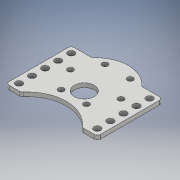
# Autodesk Inventor part: NeverRestMotorMount
Saved by Autodesk Inventor 2018 (Build 220112000, 112)
## iProperties
Created: 2017-11-21
Part Number: NeverRestMotorMount
Material: Generic
Document SubType Name: Modeling
Designer: JM_MRI
Density: 1 g/cm^3
Appearance: Default
Author: JM_MRI
Autodesk Inventor part; units mm, degrees
ref_plane "YZ Plane" through (0, 0, 0) normal (1, 0, 0) x (0, 1, 0)
ref_plane "XZ Plane" through (0, 0, 0) normal (0, 1, 0) x (-1, 0, 0)
ref_plane "XY Plane" through (0, 0, 0) normal (0, 0, 1) x (1, 0, 0)
sketch "Sketch1" plane through (0, 0, 0) normal (0, 0, 1) x (1, 0, 0)
  line L0 (56, 0) -> (56, 40)
  line L1 (0, 40) -> (0, 0)
  circle A0 centre (28, 20) radius 6.1
  circle A1 centre (43.5, 27) radius 1.75
  circle A2 centre (35.75, 40.4234) radius 1.75
  circle A3 centre (20.25, 40.4234) radius 1.75
  circle A4 centre (12.5, 27) radius 1.75
  circle A5 centre (20.25, 13.5766) radius 1.75
  circle A6 centre (35.75, 13.5766) radius 1.75
  arc A7 (43.1987, 40) -> (12.8013, 40) centre (28, 27) ccw
  line L2 (56, 40) -> (43.1987, 40)
  line L3 (12.8013, 40) -> (0, 40)
  circle A8 centre (4, 36) radius 2.05
  circle A9 centre (4, 28) radius 2.05
  circle A10 centre (4, 20) radius 2.05
  circle A11 centre (4, 12) radius 2.05
  circle A12 centre (4, 4) radius 2.05
  circle A13 centre (52, 36) radius 2.05
  circle A14 centre (52, 28) radius 2.05
  circle A15 centre (52, 20) radius 2.05
  circle A16 centre (52, 12) radius 2.05
  circle A17 centre (52, 4) radius 2.05
  arc A18 (46.735, 0) -> (9.265, 0) centre (28, -15) ccw
  line L4 (0, 0) -> (9.265, 0)
  line L5 (46.735, 0) -> (56, 0)
  dimension "d0" = 40
  dimension "d1" = 56
  dimension "d2" = 12.2
  dimension "d4" = 28
  dimension "d5" = 7
  dimension "d6" = 15.5
  dimension "d7" = 3.5
  dimension "d10" = 360
  dimension "d12" = 20
  dimension "d14" = 20
  dimension "d15" = 4.1
  dimension "d16" = 4
  dimension "d17" = 4
  dimension "d20" = 8
  dimension "d23" = 48
  dimension "d26" = 28
  dimension "d28" = 24
  dimension "d29" = 15
  constraints: 19 centre point, 12 end point, 5 parallel, 4 point on circle, 3 horizontal, 3 horizontal alignment, 2 perpendicular, 1 coincident, 1 vertical, 1 vertical alignment, 31 other
  measures "d0" distance of L1.start L1.end
  measures "d1" distance of L0.end L1.start
  measures "d2" diameter of A0
  measures "d4" distance from line of L1 A0.centre
  measures "d5" distance of A0.centre point (28, 27)
  measures "d6" distance of point (28, 27) A1.centre
  measures "d7" diameter of A1
  measures "d12" radius of A7
  measures "d14" distance from line of L3 A0.centre
  measures "d15" diameter of A8
  measures "d16" distance from line of L1 A8.centre
  measures "d17" distance from line of L3 A8.centre
  measures "d20" distance of A8.centre A9.centre
  measures "d23" distance of A8.centre A13.centre
  measures "d26" distance from line of L1 A18.centre
  measures "d28" radius of A18
  measures "d29" distance from line of L4 A18.centre
extrude "Extrusion1" add sketch "Sketch1" against normal blind 2.5
fillet "Fillet1" radius 2 6 edges at (0, 40, -1.25) (0, 0, -1.25) (56, 0, -1.25) (56, 40, -1.25) (9.265, 0, -1.25) (46.735, 0, -1.25)
body "Solid1"
